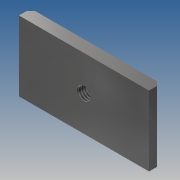
# Autodesk Inventor part: DD_KVD_004_04_B
Saved by Autodesk Inventor 2017.3 (Build 213256000, 256)
## iProperties
Created: 2023-11-02
Part Number: DD_KVD_004_04_B
Material: Nerezová ocel
Document SubType Name: Sheet Metal
Designer: Darena
Density: 8 g/cm^3
Sheet Metal Rule: Výchozí_mm
Appearance: Pololeštěná
Flat Pattern Width: 3.5 cm
Flat Pattern Length: 6.5 cm
Flat Pattern Area: 22.75 cm^2
Sheet Metal Width: 35,000 mm
Sheet Metal Length: 65,000 mm
Sheet Metal Area: 2275,000 mm^2
Author: Darena
Autodesk Inventor part; units mm, degrees
ref_plane "YZ Plane" through (0, 0, 0) normal (1, 0, 0) x (0, 1, 0)
ref_plane "XZ Plane" through (0, 0, 0) normal (0, 1, 0) x (-1, 0, 0)
ref_plane "XY Plane" through (0, 0, 0) normal (0, 0, 1) x (1, 0, 0)
sketch "Náčrt2" plane through (0, 0, 0) normal (0, 1, 0) x (-1, 0, 0)
  line L0 (32.5, 17.5) -> (-32.5, 17.5)
  line L1 (-32.5, 17.5) -> (-32.5, -17.5)
  line L2 (-32.5, -17.5) -> (32.5, -17.5)
  line L3 (32.5, -17.5) -> (32.5, 17.5)
  point P0 (0, 0)
  point P1 (32.5, 0)
  point P2 (0, 17.5)
  dimension "d0" = 65
  dimension "d1" = 35
  constraints: 8 end point, 2 midpoint, 2 parallel, 1 horizontal, 1 horizontal alignment, 1 perpendicular, 1 vertical alignment
  measures "d0" distance of L0.start L0.end
  measures "d1" distance of L2.end L0.start
extrude "Vysunutí1" add sketch "Náčrt2" along normal blind 6
chamfer "Zkosení3" distance 2 angle 45 2 edges at (-32.5, 6, 0) (32.5, 6, 0)
sketch "Náčrt6" plane through (0, 6, 0) normal (0, 1, 0) x (1, 0, 0)
  point P0 (0, 0)
hole "Díra1" at (0, 6, 0) direction (0, -1, 0) diameter 6.647 end through all thread size "M8x1.25" class "6H" standard "ISO Metric profile"
chamfer "Zkosení4" distance 0.4 angle 45 1 edges at (0, 6, -3.3235)
equation "\"PoloměrOhybu\" = Tloušťka"
equation "\"ŠířkaVýštipu\" = Tloušťka"
equation "\"HloubkaVýštipu\" = 0.5 * Tloušťka"
equation "\"MinimálníZbytek\" = 2 * Tloušťka"
equation "\"PřechodovýPoloměr\" = PoloměrOhybu"
equation "\"VelikostJacobihoPoloměru\" = PoloměrOhybu"
equation "\"VelikostMezery\" = Tloušťka"
equation "\"Tloušťka\" = 2.5"
